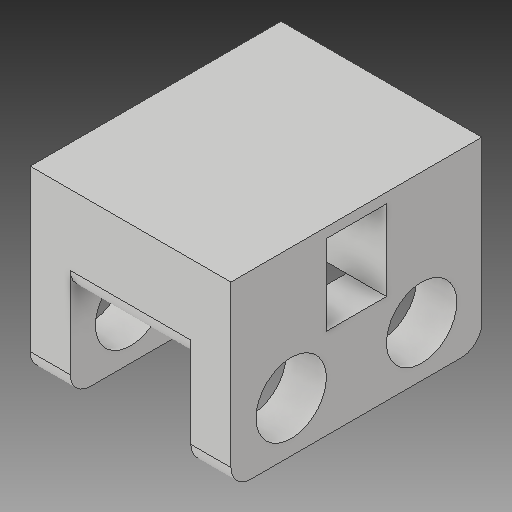
# Autodesk Inventor part: Salida
Saved by Autodesk Inventor 2019 (Build 230136000, 136)
## iProperties
Created: 2020-02-05
Part Number: Salida
Material: Generic
Document SubType Name: Modeling
Designer: Elías Sánchez
Density: 1 g/cm^3
Appearance: Default
Description: Impresión 3D
Author: Elías Sánchez
Autodesk Inventor part; units mm, degrees
ref_plane "YZ Plane" through (0, 0, 0) normal (1, 0, 0) x (0, 1, 0)
ref_plane "XZ Plane" through (0, 0, 0) normal (0, 1, 0) x (-1, 0, 0)
sketch "Sketch1" plane through (0, 0, 0) normal (0, 0, 1) x (1, 0, 0)
  line L0 (20, 0) -> (20, 18)
  line L1 (20, 18) -> (0, 18)
  line L2 (0, 18) -> (0, 0)
  line L3 (0, 0) -> (4, 0)
  line L4 (4, 0) -> (4, 9)
  line L5 (4, 9) -> (16, 9)
  line L6 (16, 9) -> (16, 0)
  line L7 (16, 0) -> (20, 0)
  point P0 (10, 9)
  point P1 (10, 18)
  dimension "d0" = 18
  dimension "d1" = 20
  dimension "d2" = 9
  dimension "d28" = 12
  dimension "d29" = 4
  dimension "d30" = 4
  constraints: 16 end point, 4 perpendicular, 2 midpoint, 1 horizontal, 1 parallel, 1 point on line, 1 vertical alignment
  measures "d0" distance of L0.start L0.end
  measures "d1" distance of L0.end L1.end
  measures "d2" distance of L3.end L4.end
  measures "d28" distance of L4.end L5.end
  measures "d29" distance of L2.end L3.end
  measures "d30" distance of L6.end L0.start
extrude "Extrusion1" add sketch "Sketch1" along normal blind 25
sketch "Sketch2" plane through (0, 0, 0) normal (-1, 0, 0) x (0, 0, 1)
  line L0 (0, 0) -> (25, 0) projected
  line L1 (0, 0) -> (0, 18) projected
  point P0 (6, 5)
  dimension "d10" = 5
  dimension "d11" = 6
  measures "d10" distance from line of L0 point (6, 5)
  measures "d11" distance from line of L1 point (6, 5)
hole "Hole1" at (0, 5, 6) direction (1, 0, 0) diameter 7 end through all
ref_plane "Work Plane1" through (0, 0, 12.5) normal (0, 0, 1) x (1, 0, 0)
mirror "Mirror1" about plane through (0, 0, 12.5) normal (0, 0, 1) of "Hole1"
fillet "Fillet1" radius 2 6 edges at (10, 9, 0) (2, 0, 0) (18, 0, 0) (2, 0, 25) (18, 0, 25) (10, 9, 25)
sketch "Sketch3" plane through (20, 18, 25) normal (1, 0, 0) x (0, 0, -1)
  line L0 (9.5, -1) -> (15.5, -1)
  line L1 (15.5, -1) -> (15.5, -9)
  line L2 (15.5, -9) -> (9.5, -9)
  line L3 (9.5, -9) -> (9.5, -1)
  line L4 (25, 0) -> (0, 0) projected
  line L5 (0, -16) -> (0, 0) projected
  point P0 (25, -18)
  dimension "d21" = 6
  dimension "d22" = 8
  dimension "d24" = 9
  dimension "d25" = 9.5
  constraints: 8 end point, 2 parallel, 1 horizontal, 1 perpendicular
  measures "d21" distance of L1.end L2.end
  measures "d22" distance of L0.end L1.end
  measures "d24" distance between parallel lines of L4 L2
  measures "d25" distance between parallel lines of L5 L3
extrude "Extrusion2" cut sketch "Sketch3" against normal blind 20
body "Solid1"
